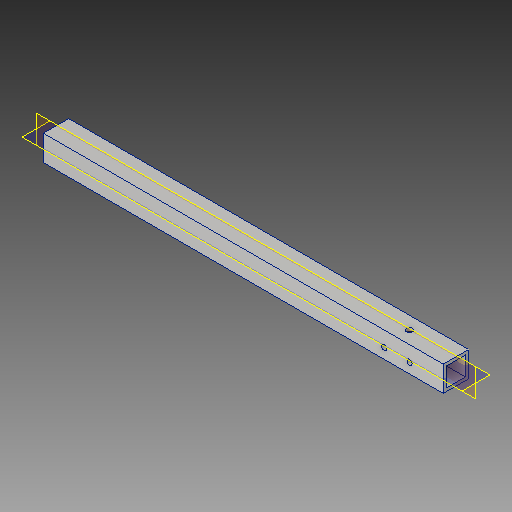
# Autodesk Inventor part: Large crossbeam
Saved by Autodesk Inventor 2017 (Build 210142000, 142)
## iProperties
Created: 2016-09-25
Part Number: Large crossbeam
Material: Aluminum 6061
Document SubType Name: Sheet Metal
Designer: Hanson
Density: 2.7 g/cm^3
Sheet Metal Rule: Default
Appearance: Aluminum - Flat
Mass: 303.616 g
Surface Area: 717.32 cm^2
Volume: 112.45 cm^3
Author: Hanson
Autodesk Inventor part; units mm, degrees
ref_plane "YZ Plane" through (0, 0, 0) normal (1, 0, 0) x (0, 1, 0)
ref_plane "XZ Plane" through (0, 0, 0) normal (0, 1, 0) x (-1, 0, 0)
sketch "Sketch1" plane through (0, 0, 0) normal (0, 1, 0) x (-1, 0, 0)
  line L0 (0, 0) -> (-400.05, 0)
  line L1 (-400.05, 0) -> (-400.05, -25.4)
  line L2 (-400.05, -25.4) -> (0, -25.4)
  line L3 (0, -25.4) -> (0, 0)
  dimension "d0" = 400.05
  dimension "d1" = 25.4
  constraints: 8 end point, 2 parallel, 1 horizontal, 1 perpendicular
  measures "d0" distance of L2.end L1.end
  measures "d1" distance of L0.end L1.end
extrude "Extrusion1" add sketch "Sketch1" along normal blind 3.175
ref_plane "Work Plane1" through (200.025, 0, 0) normal (1, 0, 0) x (0, 0, -1)
sketch "Sketch7" plane through (0, 3.175, 0) normal (0, 1, 0) x (1, 0, 0)
  line L0 (400.05, 0) -> (400.05, 25.4) projected
  line L1 (0, 0) -> (400.05, 0)
  line L2 (400.05, 0) -> (400.05, 3.175)
  line L3 (400.05, 3.175) -> (0, 3.175)
  line L4 (0, 3.175) -> (0, 0)
  dimension "d49" = 3.175
  constraints: 8 end point, 2 parallel, 1 horizontal, 1 perpendicular, 1 point on line
  measures "d49" distance of L2.end L1.end
extrude "Extrusion2" add sketch "Sketch7" along normal blind 22.225
ref_plane "Work Plane2" through (0, 0, -12.7) normal (0, 0, 1) x (1, 0, 0)
mirror "Mirror2" about plane through (0, 0, -12.7) normal (0, 0, 1) of "Extrusion2"
sketch "Sketch8" plane through (0, 3.175, -22.225) normal (0, 0, 1) x (1, 0, 0)
  line L0 (400.05, 22.225) -> (0, 22.225) projected
  line L1 (400.05, 22.225) -> (0, 22.225)
  line L2 (0, 22.225) -> (0, 19.05)
  line L3 (0, 19.05) -> (400.05, 19.05)
  line L4 (400.05, 19.05) -> (400.05, 22.225)
  point P0 (0, -3.175)
  dimension "d52" = 400.05
  dimension "d53" = 3.175
  constraints: 8 end point, 2 parallel, 1 horizontal, 1 perpendicular
  measures "d52" distance of L3.end L2.end
  measures "d53" distance of L2.end L1.end
extrude "Extrusion3" add sketch "Sketch8" along normal blind 19.05
ref_plane "Work Plane3" through (0, 12.7, 0) normal (0, -1, 0) x (1, 0, 0)
sketch "Sketch10" plane through (400.05, 0, -25.4) normal (0, 0, -1) x (-1, 0, 0)
  line L0 (0, 0) -> (400.05, 0) projected
  line L1 (0, 0) -> (0, 25.4) projected
  point P0 (59.0956, 10.1854)
  dimension "d61" = 10.1854
  dimension "d62" = 59.0956
  measures "d61" distance from line of L0 point (59.096, 10.185)
  measures "d62" distance from line of L1 point (59.096, 10.185)
sketch "Sketch11" plane through (400.05, 0, -25.4) normal (0, 0, -1) x (-1, 0, 0)
  line L0 (0, 0) -> (400.05, 0) projected
  line L1 (0, 0) -> (0, 25.4) projected
  point P0 (33.6956, 10.1854)
  dimension "d70" = 10.1854
  dimension "d71" = 33.6956
  measures "d70" distance from line of L0 point (33.696, 10.185)
  measures "d71" distance from line of L1 point (33.696, 10.185)
hole "Hole8" at (340.9544, 10.1854, -25.4) direction (0, 0, 1) diameter 5.1594 end through all
hole "Hole9" at (366.3544, 10.1854, -25.4) direction (0, 0, 1) diameter 5.1594 end through all
sketch "Sketch14" plane through (0, 0, 0) normal (0, -1, 0) x (1, 0, 0)
  line L0 (400.05, 0) -> (400.05, -25.4) projected
  line L1 (400.05, -25.4) -> (0, -25.4) projected
  point P0 (0, 0)
  point P1 (353.6442, -12.7)
  dimension "d97" = 46.4058
  dimension "d98" = 12.7
  measures "d97" distance from line of L0 point (353.644, -12.7)
  measures "d98" distance from line of L1 point (353.644, -12.7)
hole "Hole10" at (353.6442, 0, -12.7) direction (0, 1, 0) diameter 6.35 end through all
equation "\"d84\" = Thickness"
equation "\"d91\" = Thickness"
equation "\"d104\" = Thickness"
equation "\"BendRadius\" = Thickness"
equation "\"BendReliefWidth\" = Thickness"
equation "\"BendReliefDepth\" = 0.5 * Thickness"
equation "\"CornerReliefSize\" = 4 * Thickness"
equation "\"MinimumRemnant\" = 2 * Thickness"
equation "\"TransitionRadius\" = BendRadius"
equation "\"JacobiRadiusSize\" = BendRadius"
equation "\"GapSize\" = Thickness"
equation "\"Thickness\" = 3.048"
body "Solid1"
